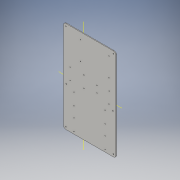
# Autodesk Inventor part: darla-board
Saved by Autodesk Inventor 2016 (Build 200138000, 138)
## iProperties
Created: 2018-01-29
Part Number: darla-board
Material: Generic
Document SubType Name: Modeling
Designer: Student
Density: 1 g/cm^3
Appearance: Default
Author: Student
Autodesk Inventor part; units mm, degrees
ref_plane "YZ Plane" through (0, 0, 0) normal (1, 0, 0) x (0, 1, 0)
ref_plane "XZ Plane" through (0, 0, 0) normal (0, 1, 0) x (-1, 0, 0)
ref_plane "XY Plane" through (0, 0, 0) normal (0, 0, 1) x (1, 0, 0)
sketch "Sketch1" plane through (0, 0, 0) normal (0, 0, 1) x (1, 0, 0)
  line L0 (0, -274.3238) -> (0, 275.9818) projected
  line L1 (-128.8749, 0) -> (188.1669, 0) projected
  line L2 (-68.779, 176.2125) -> (128.071, 176.2125) construction
  line L3 (128.071, 176.2125) -> (128.071, 79.6925) construction
  line L4 (128.071, 79.6925) -> (-68.779, 79.6925) construction
  line L5 (-68.779, 79.6925) -> (-68.779, 176.2125) construction
  line L6 (-76.399, 47.9425) -> (8.601, 47.9425) construction
  line L7 (8.601, 47.9425) -> (8.601, -8.0575) construction
  line L8 (8.601, -8.0575) -> (-76.399, -8.0575) construction
  line L9 (-76.399, -8.0575) -> (-76.399, 47.9425) construction
  line L10 (59.491, 41.5925) -> (128.071, 41.5925) construction
  line L11 (128.071, 41.5925) -> (128.071, -11.7475) construction
  line L12 (128.071, -11.7475) -> (59.491, -11.7475) construction
  line L13 (59.491, -11.7475) -> (59.491, 41.5925) construction
  line L14 (-39.139, -37.1475) -> (98.861, -37.1475) construction
  line L15 (98.861, -37.1475) -> (98.861, -93.1475) construction
  line L16 (98.861, -93.1475) -> (-39.139, -93.1475) construction
  line L17 (-39.139, -93.1475) -> (-39.139, -37.1475) construction
  line L18 (-71.319, 195.2625) -> (130.611, 195.2625)
  line L19 (140.771, 185.1025) -> (140.771, -183.4445)
  line L20 (130.611, -193.6045) -> (-71.319, -193.6045)
  line L21 (-81.479, -183.4445) -> (-81.479, 185.1025)
  arc A0 (-71.319, 195.2625) -> (-81.479, 185.1025) centre (-71.319, 185.1025) ccw
  arc A1 (140.771, 185.1025) -> (130.611, 195.2625) centre (130.611, 185.1025) ccw
  arc A2 (130.611, -193.6045) -> (140.771, -183.4445) centre (130.611, -183.4445) ccw
  arc A3 (-81.479, -183.4445) -> (-71.319, -193.6045) centre (-71.319, -183.4445) ccw
  line L22 (-39.1372, -131.2475) -> (98.861, -131.2475) construction
  line L23 (98.861, -131.2475) -> (98.861, -187.2545) construction
  line L24 (98.861, -187.2545) -> (-39.1372, -187.2545) construction
  line L25 (-39.1372, -187.2545) -> (-39.1372, -131.2475) construction
  circle A4 centre (-8.4286, 87.5665) radius 1.524
  circle A5 centre (-8.4286, 167.5765) radius 1.524
  circle A6 centre (111.561, 87.5665) radius 1.524
  circle A7 centre (111.561, 167.5765) radius 1.524
  circle A8 centre (-52.8872, 44.4391) radius 1.524
  circle A9 centre (5.101, 44.4391) radius 1.524
  circle A10 centre (-52.8872, -4.5575) radius 1.524
  circle A11 centre (5.101, -4.5575) radius 1.524
  circle A12 centre (60.761, 33.9725) radius 1.524
  circle A13 centre (112.831, 39.0525) radius 1.524
  circle A14 centre (60.761, 6.0325) radius 1.524
  circle A15 centre (111.561, -9.2075) radius 1.524
  circle A16 centre (-36.599, -39.6875) radius 1.524
  circle A17 centre (-36.599, -89.5985) radius 1.524
  circle A18 centre (95.4048, -39.6875) radius 1.524
  circle A19 centre (95.4048, -89.5985) radius 1.524
  circle A20 centre (-36.5972, -133.7875) radius 1.524
  circle A21 centre (-36.5972, -183.6985) radius 1.524
  circle A22 centre (95.4066, -133.7875) radius 1.524
  circle A23 centre (95.4066, -183.6985) radius 1.524
  circle A24 centre (-71.319, 185.1025) radius 2.032
  circle A25 centre (130.611, 185.1025) radius 2.032
  circle A26 centre (-71.319, -183.4515) radius 2.032
  circle A27 centre (130.611, -183.4515) radius 2.032
  circle A28 centre (-68.779, -25.4) radius 2.032
  circle A29 centre (128.071, -25.4) radius 2.032
  point P0 (60.761, 6.0325)
  dimension "d48" = 196.85
  dimension "d49" = 96.52
  dimension "d61" = 85
  dimension "d62" = 56
  dimension "d67" = 27.94
  dimension "d69" = 50.8
  dimension "d71" = 5.08
  dimension "d72" = 1.27
  dimension "d85" = 15.24
  dimension "d87" = 1.27
  dimension "d88" = 2.54
  dimension "d89" = 68.58
  dimension "d90" = 53.34
  dimension "d91" = 2.54
  dimension "d92" = 2.54
  dimension "d93" = 138
  dimension "d94" = 56
  dimension "d119" = 50.8
  dimension "d122" = 10.16
  dimension "d170" = 31.75
  dimension "d171" = 38.1
  dimension "d208" = 2.54
  dimension "d209" = 56.007
  dimension "d210" = 137.9982
  dimension "d212" = 3.048
  dimension "d215" = 80.01
  dimension "d218" = 119.9896
  dimension "d221" = 3.048
  dimension "d224" = 57.9882
  dimension "d227" = 48.9966
  dimension "d230" = 3.048
  dimension "d231" = 3.048
  dimension "d232" = 3.048
  dimension "d233" = 3.048
  dimension "d234" = 3.048
  dimension "d237" = 49.911
  dimension "d240" = 132.0038
  dimension "d243" = 3.048
  dimension "d246" = 49.911
  dimension "d249" = 132.0038
  dimension "d256" = 19.05
  dimension "d259" = 12.7
  dimension "d261" = 4.064
  dimension "d264" = 201.93
  dimension "d267" = 368.554
  dimension "d271" = 4.064
  dimension "d272" = 4.064
  dimension "d273" = 12.7
  dimension "d274" = 12.7
  dimension "d280" = 8.636
  dimension "d283" = 3.5
  dimension "d284" = 3.5
  dimension "d285" = 5.08
  dimension "d287" = 41.91
  dimension "d288" = 41.91
  dimension "d289" = 6.35
  dimension "d290" = 38.1
  constraints: 48 end point, 30 centre point, 12 parallel, 11 horizontal, 9 coincident, 8 point on circle, 8 tangent, 6 perpendicular, 5 vertical, 3 equal radius, 1 collinear, 30 other
  measures "d48" distance of L2.start L2.end
  measures "d49" distance of L2.end L3.end
  measures "d61" distance of L7.end L8.end
  measures "d62" distance of L6.end L7.end
  measures "d67" distance of point (60.761, 6.032) point (60.761, 33.972)
  measures "d69" horizontal distance of point (111.561, -9.208) point (60.761, 6.032)
  measures "d71" vertical distance of point (112.831, 39.052) point (60.761, 33.972)
  measures "d72" horizontal distance of point (112.831, 39.052) point (111.561, -9.208)
  measures "d85" vertical distance of point (111.561, -9.208) point (60.761, 6.032)
  measures "d87" distance from line of L13 point (60.761, 33.972)
  measures "d88" distance from line of L10 point (112.831, 39.052)
  measures "d89" distance of L10.start L10.end
  measures "d90" distance of L10.end L11.end
  measures "d91" distance from line of L14 point (-36.599, -39.688)
  measures "d92" distance from line of L17 point (-36.599, -39.688)
  measures "d93" distance of L14.start L14.end
  measures "d94" distance of L14.end L15.end
  measures "d119" horizontal distance of point (111.561, -9.208) point (60.761, 33.972)
  measures "d122" radius of A0
  measures "d170" distance between parallel lines of L4 L6
  measures "d171" distance between parallel lines of L4 L10
  measures "d208" distance from line of L25 point (-36.597, -133.788)
  measures "d209" distance of L22.end L23.end
  measures "d210" distance of L23.end L24.end
  measures "d212" diameter of A4
  measures "d215" distance of A4.centre A5.centre
  measures "d218" distance of A4.centre A6.centre
  measures "d221" diameter of A8
  measures "d224" distance of A8.centre A9.centre
  measures "d227" distance of A8.centre A10.centre
  measures "d230" diameter of A12
  measures "d231" diameter of A13
  measures "d232" diameter of A14
  measures "d233" diameter of A15
  measures "d234" diameter of A16
  measures "d237" distance of A16.centre A17.centre
  measures "d240" distance of A16.centre A18.centre
  measures "d243" diameter of A20
  measures "d246" distance of A20.centre A21.centre
  measures "d249" distance of A20.centre A22.centre
  measures "d256" distance between parallel lines of L18 L2
  measures "d259" distance between parallel lines of L21 L5
  measures "d261" diameter of A24
  measures "d264" distance of A24.centre A25.centre
  measures "d267" distance of A24.centre A26.centre
  measures "d271" diameter of A28
  measures "d272" diameter of A29
  measures "d273" distance from line of L19 A29.centre
  measures "d274" distance from line of L21 A28.centre
  measures "d280" distance from line of L2 A7.centre
  measures "d283" distance from line of L7 A11.centre
  measures "d284" distance from line of A11.centre L8
  measures "d285" distance between parallel lines of L21 L9
  measures "d287" distance between parallel lines of L19 L23
  measures "d288" distance between parallel lines of L19 L15
  measures "d289" distance between parallel lines of L20 L24
  measures "d290" distance between parallel lines of L22 L16
extrude "Extrusion3" add sketch "Sketch1" along normal blind 3.175
body "Solid3"
